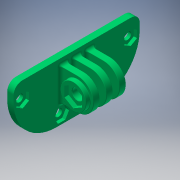
# Autodesk Inventor part: camera_bracket_female
Saved by Autodesk Inventor 2018 (Build 220112000, 112)
## iProperties
Created: 2018-06-20
Part Number: camera_bracket_female
Material: Generic
Document SubType Name: Modeling
Designer: car
Mass: 9.04679 g
Surface Area: 61.732 cm^2
Volume: 8.53471 cm^3
Density: 1 g/cm^3
Appearance: Default
iToolsLastSavedTime: 26-06-2018 09:38:27
iToolsLastSavedBy: car
iToolsMass: 0,000
LastSavedDate: 26-06-2018
LastSavedTime: 09:38:27
LastSavedBy: CAR
Reserved: False
Title: =<Part number>
Author: car
## iProperties of the stored document platform_mount_3DPrint.ipt
Created: 2019-10-08
Part Number: platform_mount_3DPrint
Material: Generic
Document SubType Name: Modeling
Designer: ZEUSLAP
Density: 1 g/cm^3
Appearance: Default
Author: ZEUSLAP
Autodesk Inventor part; units mm, degrees
ref_plane "YZ Plane" through (0, 0, 0) normal (1, 0, 0) x (0, 1, 0)
sketch "Sketch1" plane through (0, 0, 0) normal (0, 0, 1) x (1, 0, 0)
  circle A0 centre (0, 0) radius 7.5
  circle A1 centre (0, 0) radius 2.5
  line L0 (-7.5, -8) -> (7.5, -8)
  line L1 (7.5, -8) -> (7.5, 0)
  line L2 (-7.5, -8) -> (-7.5, 0)
  point P0 (0, -8)
  dimension "d2" = 15
  dimension "d3" = 5
  dimension "d6" = 8
  constraints: 6 end point, 2 centre point, 2 coincident, 2 point on circle, 2 tangent, 1 horizontal, 1 midpoint, 1 vertical alignment
  measures "d2" diameter of A0
  measures "d3" diameter of A1
  measures "d6" distance from line of L0 point (0, 0)
extrude "Extrusion2" add sketch "Sketch1" along normal mid plane 3
ref_plane "Work Plane1" through (0, 0, 4.6) normal (0, 0, 1) x (1, 0, 0)
ref_plane "Work Plane2" through (0, 0, -4.6) normal (0, 0, 1) x (1, 0, 0)
ref_plane "Work Plane3" through (0, 0, 7.6) normal (0, 0, 1) x (1, 0, 0)
ref_plane "Work Plane4" through (0, 0, -7.6) normal (0, 0, 1) x (1, 0, 0)
extrude "Extrusion3" add sketch "Sketch1" against normal up to surface (3 mm away) from surface at -4.6
extrude "Extrusion4" add sketch "Sketch1" along normal up to surface (3 mm away) from surface at 4.6
fillet "Fillet2" radius 0.2 10 edges at (0, 7.5, 7.6) (0, 7.5, -7.6) (0, 7.5, -4.6) (-7.5, -4, -1.5) (0, 7.5, -1.5) (7.5, -4, -1.5) (0, 7.5, 1.5) (-7.5, -4, 1.5) (0, 7.5, 4.6) (7.5, -4, 1.5)
sketch "Sketch4" plane through (0, 0, -7.6) normal (0, 0, -1) x (-1, 0, 0)
  circle A0 centre (0, 0) radius 2.5 projected
  line L0 (2.3671, 4.1) -> (4.7343, 0)
  line L1 (4.7343, 0) -> (2.3671, -4.1)
  line L2 (2.3671, -4.1) -> (-2.3671, -4.1)
  line L3 (-2.3671, -4.1) -> (-4.7343, 0)
  line L4 (-4.7343, 0) -> (-2.3671, 4.1)
  line L5 (-2.3671, 4.1) -> (2.3671, 4.1)
  circle A1 centre (0, 0) radius 6
  dimension "d28" = 8.2
  dimension "d29" = 12
  constraints: 12 end point, 2 coincident, 1 centre point, 13 other
  measures "d28" distance between parallel lines of L2 L5
  measures "d29" diameter of A1
extrude "Extrusion7" add sketch "Sketch4" along normal blind 2 contours A1
fillet "Fillet3" radius 0.2 2 edges at (6, 0, -7.6) (6, 0, -9.6)
chamfer "Chamfer1" distance 0.2 angle 45 6 edges at (-2.5, 0, -4.6) (-2.5, 0, -7.6) (-2.5, 0, -1.5) (-2.5, 0, 4.6) (-2.5, 0, 1.5) (-2.5, 0, 7.6)
sketch "bottom sketch" plane through (-7.3, -8, 7.6) normal (0, -1, 0) x (1, 0, 0)
  line L0 (10.8, 21.9) -> (17.8, 21.9)
  line L1 (17.8, 21.9) -> (17.8, -37.1)
  line L2 (17.8, -37.1) -> (10.8, -37.1)
  line L3 (-9.2, -17.1) -> (-9.2, 1.9)
  circle A0 centre (9.8, 17.65) radius 1.75
  circle A1 centre (9.8, -32.85) radius 1.75
  circle A2 centre (-5.2, -0.6) radius 1.75
  circle A3 centre (-5.2, -14.6) radius 1.75
  line L4 (26.7849, -7.6) -> (-19.4904, -7.6) construction
  line L5 (-0.2, -2.8) -> (-0.2, -0.2) projected
  line L6 (1.8, 7.4) -> (5.8, 7.4)
  line L7 (5.8, 7.4) -> (5.8, -22.6)
  line L8 (5.8, -22.6) -> (1.8, -22.6)
  line L9 (1.8, -22.6) -> (1.8, 7.4)
  arc A4 (-9.2, -17.1) -> (10.8, -37.1) centre (10.8, -17.1) ccw
  arc A5 (10.8, 21.9) -> (-9.2, 1.9) centre (10.8, 1.9) ccw
  point P0 (7.3, -7.6)
  point P1 (-9.2, 21.9)
  point P2 (-9.2, -37.1)
  point P3 (-9.2, -7.6)
  point P4 (5.8, -7.6)
  dimension "d57" = 59
  dimension "d58" = 27
  dimension "d59" = 3.5
  dimension "d60" = 50.5
  dimension "d61" = 14
  dimension "d62" = 15
  dimension "d63" = 4
  dimension "d66" = 5
  dimension "d69" = 4
  dimension "d70" = 30
  dimension "d71" = 7
  dimension "d72" = 20
  constraints: 18 end point, 6 centre point, 5 point on line, 4 equal radius, 4 parallel, 4 point on circle, 4 tangent, 3 horizontal, 2 horizontal alignment, 2 midpoint, 2 perpendicular, 2 vertical alignment, 2 other
  measures "d57" distance of L0.end L1.end
  measures "d58" distance of point (-9.2, 21.9) L0.end
  measures "d59" diameter of A2
  measures "d60" distance of A0.centre A1.centre
  measures "d61" distance of A2.centre A3.centre
  measures "d62" horizontal distance of A3.centre A1.centre
  measures "d63" distance from line of L3 A3.centre
  measures "d66" distance from line of L5 A2.centre
  measures "d69" distance of L7.end L8.end
  measures "d70" distance of L6.end L7.end
  measures "d71" distance from line of L9 A3.centre
  measures "d72" radius of A4
extrude "bottom" add sketch "bottom sketch" along normal blind 3 contours L0 L1 L2 A4 L3 A5 | L6 L7 L8 L9
fillet "Fillet11" radius 4 2 edges at (10.5, -9.5, -29.5) (10.5, -9.5, 29.5)
fillet "Fillet12" radius 1.5 24 edges at (-7.4414, -8, -7.5414) (0, -8, -7.6) (7.4414, -8, -7.5414) (7.5, -8, -6.1) (7.4414, -8, -4.6586) (0, -8, -4.6) (-7.4414, -8, -4.6586) (-7.5, -8, -6.1) (-7.4414, -8, -1.4414) (0, -8, -1.5) (7.4414, -8, -1.4414) (7.5, -8, 0) (7.4414, -8, 1.4414) (0, -8, 1.5) (-7.4414, -8, 1.4414) (-7.5, -8, 0) (-7.4414, -8, 7.5414) (0, -8, 7.6) (7.4414, -8, 7.5414) (7.5, -8, 6.1) (7.4414, -8, 4.6586) (0, -8, 4.6) (-7.4414, -8, 4.6586) (-7.5, -8, 6.1)
sketch "Sketch9" plane through (-7.3, -8, 7.6) normal (0, 1, 0) x (1, 0, 0)
  circle A0 centre (9.8, 32.85) radius 1.75 projected
  circle A1 centre (-5.2, 14.6) radius 1.75 projected
  circle A2 centre (9.8, -17.65) radius 1.75 projected
  circle A3 centre (-5.2, 0.6) radius 1.75 projected
  circle A4 centre (9.8, 32.85) radius 1.75 projected
  line L0 (11.5321, 29.85) -> (8.0679, 29.85)
  line L1 (8.0679, 29.85) -> (6.3359, 32.85)
  line L2 (6.3359, 32.85) -> (8.0679, 35.85)
  line L3 (8.0679, 35.85) -> (11.5321, 35.85)
  line L4 (11.5321, 35.85) -> (13.2641, 32.85)
  line L5 (13.2641, 32.85) -> (11.5321, 29.85)
  line L6 (-8.2, 12.8679) -> (-8.2, 16.3321)
  line L7 (-8.2, 16.3321) -> (-5.2, 18.0641)
  line L8 (-5.2, 18.0641) -> (-2.2, 16.3321)
  line L9 (-2.2, 16.3321) -> (-2.2, 12.8679)
  line L10 (-2.2, 12.8679) -> (-5.2, 11.1359)
  line L11 (-5.2, 11.1359) -> (-8.2, 12.8679)
  line L12 (-8.2, 2.3321) -> (-5.2, 4.0641)
  line L13 (-5.2, 4.0641) -> (-2.2, 2.3321)
  line L14 (-2.2, 2.3321) -> (-2.2, -1.1321)
  line L15 (-2.2, -1.1321) -> (-5.2, -2.8641)
  line L16 (-5.2, -2.8641) -> (-8.2, -1.1321)
  line L17 (-8.2, -1.1321) -> (-8.2, 2.3321)
  line L18 (13.2641, -17.65) -> (11.5321, -20.65)
  line L19 (11.5321, -20.65) -> (8.0679, -20.65)
  line L20 (8.0679, -20.65) -> (6.3359, -17.65)
  line L21 (6.3359, -17.65) -> (8.0679, -14.65)
  line L22 (8.0679, -14.65) -> (11.5321, -14.65)
  line L23 (11.5321, -14.65) -> (13.2641, -17.65)
  point P0 (7.3, 7.6)
  point P1 (-1.7, 13.6986)
  point P2 (-1.6495, 15.4114)
  point P3 (-1.6495, -0.2114)
  point P4 (-1.7, 1.5014)
  dimension "d73" = 6
  constraints: 48 end point, 4 coincident, 3 equal length, 2 horizontal, 2 vertical, 54 other
  measures "d73" distance between parallel lines of L0 L3
extrude "Extrusion12" cut sketch "Sketch9" against normal blind 1.5 contours A1 | A3 | L0 L1 L2 L3 L4 L5 | L6 L7 L8 L9 L10 L11 | L12 L13 L14 L15 L16 L17 | L18 L19 L20 L21 L22 L23
body "Solid2"
